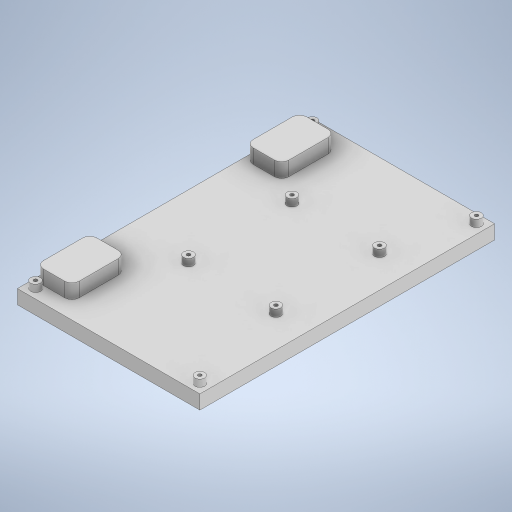
# Autodesk Inventor part: wisecoco-display
Saved by Autodesk Inventor 2024 (Build 280153000, 153)
## iProperties
Created: 2024-08-25
Part Number: wisecoco-display
Material: Generic
Document SubType Name: Modeling
Designer: Stefano
Density: 1 g/cm^3
Appearance: Default
Author: Stefano
Autodesk Inventor part; units mm, degrees
ref_plane "YZ Plane" through (0, 0, 0) normal (1, 0, 0) x (0, 1, 0)
ref_plane "XZ Plane" through (0, 0, 0) normal (0, 1, 0) x (-1, 0, 0)
ref_plane "XY Plane" through (0, 0, 0) normal (0, 0, 1) x (1, 0, 0)
sketch "Sketch1" plane through (0, 0, 0) normal (0, 1, 0) x (-1, 0, 0)
  line L0 (51.1175, 82.55) -> (-51.1175, 82.55)
  line L1 (-51.1175, 82.55) -> (-51.1175, -82.55)
  line L2 (-51.1175, -82.55) -> (51.1175, -82.55)
  line L3 (51.1175, -82.55) -> (51.1175, 82.55)
  line L4 (51.1175, 82.55) -> (-51.1175, -82.55) construction
  line L5 (-51.1175, 82.55) -> (51.1175, -82.55) construction
  point P0 (0, 0)
  dimension "d0" = 165.1
  dimension "d1" = 102.235
  constraints: 12 end point, 2 midpoint, 2 parallel, 1 horizontal, 1 perpendicular
  measures "d0" distance of L2.end L0.start
  measures "d1" distance of L0.start L0.end
extrude "Extrusion1" add sketch "Sketch1" along normal blind 7.874
sketch "Sketch2" plane through (0, 7.874, 0) normal (0, 1, 0) x (1, 0, 0)
  circle A0 centre (-46, -77.5) radius 2.75
  line L0 (-51.1175, -82.55) -> (51.1175, -82.55) projected
  line L1 (-46, -77.5) -> (46, -77.5) construction
  line L2 (46, -77.5) -> (46, 77.5) construction
  line L3 (46, 77.5) -> (-46, 77.5) construction
  line L4 (-46, 77.5) -> (-46, -77.5) construction
  line L5 (-46, -77.5) -> (46, 77.5) construction
  line L6 (46, -77.5) -> (-46, 77.5) construction
  circle A1 centre (-46, 77.5) radius 2.75
  circle A2 centre (46, -77.5) radius 2.75
  circle A3 centre (46, 77.5) radius 2.75
  point P0 (0, 0)
  dimension "d4" = 5.5
  dimension "d6" = 5.5
  dimension "d7" = 5.5
  dimension "d8" = 5.5
  dimension "d9" = 160.5
  dimension "d10" = 97.5
  constraints: 12 end point, 4 centre point, 4 coincident, 2 midpoint, 2 parallel, 1 horizontal, 1 perpendicular
  measures "d4" diameter of A0
  measures "d6" diameter of A1
  measures "d7" diameter of A2
  measures "d8" diameter of A3
extrude "Extrusion2" add sketch "Sketch2" along normal blind 4
sketch "Sketch3" plane through (-46, 11.874, 77.5) normal (0, 1, 0) x (1, 0, 0)
  circle A0 centre (0, 0) radius 2.75 projected
  circle A1 centre (0, 155) radius 2.75 projected
  circle A2 centre (92, 155) radius 2.75 projected
  circle A3 centre (92, 0) radius 2.75 projected
  point P0 (46, 77.5)
  constraints: 4 coincident
hole "Hole1" at (-46, 11.874, 77.5) at (-46, 11.874, -77.5) at (46, 11.874, -77.5) at (46, 11.874, 77.5) direction (0, -1, 0) diameter 2.013 depth 4 tip angle 118 thread size "M2.5x0.45" class "6H" standard "ANSI Metric M Profile"
sketch "Sketch4" plane through (0, 7.874, 0) normal (0, 1, 0) x (1, 0, 0)
  line L0 (-49.3675, -73.75) -> (-29.3675, -73.75)
  line L1 (-29.3675, -73.75) -> (-29.3675, -43.75)
  line L2 (-29.3675, -43.75) -> (-49.3675, -43.75)
  line L3 (-49.3675, -43.75) -> (-49.3675, -73.75)
  line L4 (-49.3675, -73.75) -> (-29.3675, -43.75) construction
  line L5 (-29.3675, -73.75) -> (-49.3675, -43.75) construction
  line L6 (-51.1175, 82.55) -> (-51.1175, -82.55) projected
  line L7 (-51.1175, 0) -> (51.1175, 0) construction
  line L8 (51.1175, -82.55) -> (51.1175, 82.55) construction
  line L9 (-49.3675, 73.75) -> (-29.3675, 73.75)
  line L10 (-29.3675, 73.75) -> (-29.3675, 43.75)
  line L11 (-29.3675, 43.75) -> (-49.3675, 43.75)
  line L12 (-49.3675, 43.75) -> (-49.3675, 73.75)
  line L13 (-49.3675, 73.75) -> (-29.3675, 43.75) construction
  line L14 (-29.3675, 73.75) -> (-49.3675, 43.75) construction
  point P0 (0, 0)
  point P1 (-39.3675, -58.75)
  point P2 (-39.3675, 58.75)
  dimension "d20" = 30
  dimension "d21" = 20
  dimension "d22" = 1.75
  dimension "d23" = 147.5
  constraints: 26 end point, 5 symmetric about line, 4 midpoint, 2 parallel, 1 horizontal, 1 perpendicular
  measures "d20" distance of L2.end L0.start
  measures "d21" distance of L0.start L0.end
  measures "d22" distance between parallel lines of L6 L3
  measures "d23" distance between parallel lines of L9 L0
extrude "Extrusion3" add sketch "Sketch4" along normal blind 8
fillet "Fillet1" radius 4 8 edges at (-29.3675, 11.874, 73.75) (-49.3675, 11.874, 73.75) (-49.3675, 11.874, 43.75) (-29.3675, 11.874, 43.75) (-29.3675, 11.874, -43.75) (-49.3675, 11.874, -43.75) (-49.3675, 11.874, -73.75) (-29.3675, 11.874, -73.75)
sketch "Sketch5" plane through (0, 7.874, 0) normal (0, 1, 0) x (1, 0, 0)
  line L0 (-15.6325, -22.2) -> (33.3675, -22.2) construction
  line L1 (33.3675, -22.2) -> (33.3675, 35.8) construction
  line L2 (33.3675, 35.8) -> (-15.6325, 35.8) construction
  line L3 (-15.6325, 35.8) -> (-15.6325, -22.2) construction
  line L4 (-15.6325, -22.2) -> (33.3675, 35.8) construction
  line L5 (33.3675, -22.2) -> (-15.6325, 35.8) construction
  circle A0 centre (33.3675, 35.8) radius 2.75
  circle A1 centre (33.3675, -22.2) radius 2.75
  circle A2 centre (-15.6325, -22.2) radius 2.75
  circle A3 centre (-15.6325, 35.8) radius 2.75
  line L6 (51.1175, -82.55) -> (51.1175, 82.55) projected
  line L7 (51.1175, 82.55) -> (-51.1175, 82.55) projected
  line L8 (-51.1175, -82.55) -> (51.1175, -82.55) projected
  point P0 (0, 0)
  point P1 (8.8675, 6.8)
  dimension "d27" = 5.5
  dimension "d28" = 5.5
  dimension "d29" = 63.5
  dimension "d30" = 5.5
  dimension "d31" = 5.5
  dimension "d32" = 15
  dimension "d33" = 54.5
  dimension "d34" = 44
  dimension "d44" = 57.6
  constraints: 12 end point, 4 centre point, 4 coincident, 2 midpoint, 2 parallel, 1 horizontal, 1 perpendicular
  measures "d27" diameter of A0
  measures "d28" diameter of A1
  measures "d30" diameter of A2
  measures "d31" diameter of A3
  measures "d32" distance edge to line of A1 L6
  measures "d34" distance edge to line of A0 L7
  measures "d44" distance edge to line of A2 L8
extrude "Extrusion4" add sketch "Sketch5" along normal blind 4
sketch "Sketch6" plane through (-15.6325, 11.874, 22.2) normal (0, 1, 0) x (1, 0, 0)
  circle A0 centre (0, 58) radius 2.75 projected
  circle A1 centre (49, 58) radius 2.75 projected
  circle A2 centre (49, 0) radius 2.75 projected
  point P0 (15.6325, 22.2)
  point P1 (0, 0)
  constraints: 3 coincident
hole "Hole2" at (-15.6325, 11.874, 22.2) at (-15.6325, 11.874, -35.8) at (33.3675, 11.874, -35.8) at (33.3675, 11.874, 22.2) direction (0, -1, 0) diameter 2.013 depth 4 tip angle 118 thread size "M2.5x0.45" class "6H" standard "ANSI Metric M Profile"
body "Solid1"
